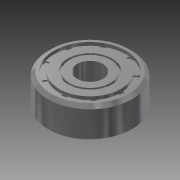
# Autodesk Inventor part: Bearing-605zz
Saved by Autodesk Inventor 2014 SP1 (Build 180222100, 222)
## iProperties
Created: 2017-05-20
Part Number: Bearing-605zz
Material: Stainless Steel
Document SubType Name: Modeling
Designer: danielsikar
Density: 8.08 g/cm^3
Appearance: Semi-Polished
Author: danielsikar
Autodesk Inventor part; units mm, degrees
ref_plane "YZ Plane" through (0, 0, 0) normal (1, 0, 0) x (0, 1, 0)
ref_plane "XZ Plane" through (0, 0, 0) normal (0, 1, 0) x (-1, 0, 0)
sketch "Sketch1" plane through (0, 0, 0) normal (0, 0, 1) x (1, 0, 0)
  circle A0 centre (0, 0) radius 6.5
  circle A1 centre (0, 0) radius 2
  dimension "d0" = 13
  dimension "d1" = 4
  constraints: 2 centre point, 2 coincident
  measures "d0" diameter of A0
  measures "d1" diameter of A1
extrude "Extrusion1" add sketch "Sketch1" along normal blind 5
chamfer "Chamfer1" distance 0.5 angle 45 2 edges at (-6.5, 0, 5) (-6.5, 0, 0)
sketch "Sketch2" plane through (0, 0, 5) normal (0, 0, 1) x (1, 0, 0)
  circle A0 centre (0, 0) radius 6 projected
  circle A1 centre (0, 0) radius 3.15
  circle A2 centre (0, 0) radius 3.45
  circle A3 centre (0, 0) radius 4.75
  circle A4 centre (0, 0) radius 5.575
  dimension "d7" = 6.3
  dimension "d8" = 6.9
  dimension "d9" = 9.5
  dimension "d10" = 11.15
  constraints: 4 centre point, 4 coincident
  measures "d7" diameter of A1
  measures "d8" diameter of A2
  measures "d9" diameter of A3
  measures "d10" diameter of A4
extrude "Extrusion2" cut sketch "Sketch2" against normal blind 0.5 contours A2 | A4
ref_plane "Work Plane1" through (0, 0, 2.5) normal (0, 0, -1) x (-1, 0, 0)
sketch "Sketch3" plane through (0, 0, 4.5) normal (0, 0, 1) x (1, 0, 0)
  circle A0 centre (0, 0) radius 4.75 projected
  circle A1 centre (0, 0) radius 5.575 projected
  circle A2 centre (0, 0) radius 4.75 construction
  circle A3 centre (0, 0) radius 5.575 construction
  line L0 (-9.1, 0) -> (9.1, 0) construction
  line L1 (4.6568, 0.35) -> (5.7132, 0.35)
  line L2 (4.5944, -0.35) -> (5.8021, -0.35)
  line L3 (5.349, 0.35) -> (5.7285, 0.35)
  arc A4 (4.7371, -0.35) -> (4.7371, 0.35) centre (0, 0) ccw
  arc A5 (5.564, -0.35) -> (5.564, 0.35) centre (0, 0) ccw
  dimension "d14" = 0.35
  dimension "d15" = 0.35
  constraints: 8 point on circle, 6 end point, 5 point on line, 3 parallel, 2 centre point
  measures "d14" distance between parallel lines of L1 L0
  measures "d15" distance between parallel lines of L2 L0
extrude "Extrusion3" cut sketch "Sketch3" against normal blind 0.2 contours A0 L1 A1 L2 picked at (5.2247, 0.1167)
pattern_circular "Circular Pattern1" count 9 over 360 about axis through (0, 0, -10) along (0, 0, 1) of "Extrusion3"
mirror "Mirror1" about plane through (0, 0, 2.5) normal (0, 0, -1) of "Circular Pattern1", "Extrusion2"
body "Solid1"
